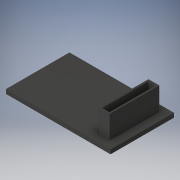
# Autodesk Inventor part: top
Saved by Autodesk Inventor 2019 (Build 230136000, 136)
## iProperties
Created: 2018-06-06
Part Number: top
Material: PBT Plastic Black
Document SubType Name: Modeling
Designer: stra92745
Density: 1.31 g/cm^3
Appearance: Smooth - White
Author: stra92745
Autodesk Inventor part; units mm, degrees
ref_plane "YZ Plane" through (0, 0, 0) normal (1, 0, 0) x (0, 1, 0)
ref_plane "XZ Plane" through (0, 0, 0) normal (0, 1, 0) x (-1, 0, 0)
ref_plane "XY Plane" through (0, 0, 0) normal (0, 0, 1) x (1, 0, 0)
sketch "Sketch1" plane through (0, 0, 0) normal (0, 1, 0) x (-1, 0, 0)
  line L0 (0, 0) -> (-99, 0)
  line L1 (-99, 0) -> (-99, -60)
  line L2 (-99, -60) -> (0, -60)
  line L3 (0, -60) -> (0, 0)
  line L4 (-83, -52) -> (-90, -52)
  line L5 (-90, -52) -> (-90, -8)
  line L6 (-90, -8) -> (-83, -8)
  line L7 (-83, -8) -> (-83, -52)
  dimension "d0" = 99
  dimension "d1" = 60
  dimension "d2" = 7
  dimension "d3" = 44
  dimension "d4" = 8
  dimension "d5" = 9
  constraints: 16 end point, 4 parallel, 2 horizontal, 2 perpendicular
  measures "d0" distance of L2.end L1.end
  measures "d1" distance of L1.end L0.end
  measures "d2" distance of L5.end L6.end
  measures "d3" distance of L6.end L4.start
  measures "d4" distance between parallel lines of L0 L6
  measures "d5" distance between parallel lines of L1 L5
extrude "Extrusion1" add sketch "Sketch1" along normal blind 4
sketch "Sketch2" plane through (0, 4, 0) normal (0, 1, 0) x (1, 0, 0)
  line L0 (83, 8) -> (83, 52) projected
  line L1 (83, 52) -> (90, 52) projected
  line L2 (90, 52) -> (90, 8) projected
  line L3 (90, 8) -> (83, 8) projected
  line L4 (91.5, 53.5) -> (81.5, 53.5)
  line L5 (81.5, 53.5) -> (81.5, 6.5)
  line L6 (81.5, 6.5) -> (91.5, 6.5)
  line L7 (91.5, 6.5) -> (91.5, 53.5)
  point P0 (0, 0)
  dimension "d8" = 1.5
  constraints: 8 end point, 3 other
  measures "d8" distance between parallel lines of L1 L4
extrude "Extrusion2" add sketch "Sketch2" along normal blind 22
body "Solid1"
